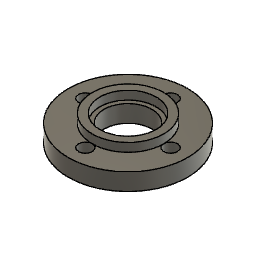
Task1 v1 (Autodesk Fusion 360 design; units mm, degrees)
Autodesk Fusion 360 part; units mm, degrees
sketch "Sketch1" plane through (0, 0, 0) normal (0, 1, 0) x (1, 0, 0)
  circle A0 centre (0, 0) radius 35
  circle A1 centre (0, 0) radius 14
  dimension "d1" = 70
  dimension "d2" = 28
  constraint coincident A0.centre A1.centre
  constraint concentric A0 A1
  measures "d1" diameter of A0
  measures "d2" diameter of A1
extrude "Extrude1" add sketch "Sketch1" along normal blind 10
sketch "Sketch2" plane through (0, 10, 0) normal (0, 1, 0) x (-1, 0, 0)
  circle A0 centre (0, 0) radius 14
  circle A1 centre (0, 0) radius 35
  circle A2 centre (0, 0) radius 16.5
  circle A3 centre (0, 0) radius 21
  circle A4 centre (0, 0) radius 25 construction
  circle A5 centre (0, -25) radius 4
  line L0 (0, 0) -> (0, -25) construction
  line L1 (0, 1.75) -> (0, 22.5)
  circle A6 centre (25, 0) radius 4
  circle A7 centre (0, 25) radius 4
  circle A8 centre (-25, 0) radius 4
  dimension "d5" = 33
  dimension "d6" = 42
  dimension "d7" = 50
  dimension "d8" = 8
  dimension "d10" = 360
  constraint concentric A0 A2
  constraint coincident A0.centre A1.centre
  constraint coincident A4 A5.centre
  constraint coincident A5.centre L0.end
  constraint parallel L0 L1
  measures "d5" diameter of A2
  measures "d6" diameter of A3
  measures "d7" diameter of A4
  measures "d8" diameter of A5
extrude "Extrude2" add sketch "Sketch2" along normal blind 5 contours A3
extrude "Extrude3" cut sketch "Sketch2" against normal blind 10 contours A5 | A8 | A7 | A6
